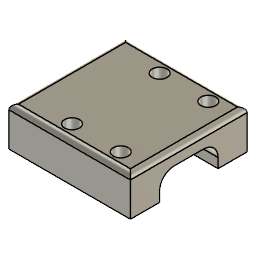
Mouse_Motor_Clamp_Upper_v3 (Autodesk Fusion 360 design; units mm, degrees)
Autodesk Fusion 360 part; units mm, degrees
note: some values were not read from the file. Set by a fixed rule: which sketch regions a step uses.
sketch "Skizze1" plane through (0, 0, 0) normal (0, 0, 1) x (1, 0, 0)
  line L0 (45, -30) -> (45, -50)
  line L1 (45, -50) -> (-45, -50)
  line L2 (-45, -50) -> (-45, -30)
  arc A0 (45, 0) -> (-45, 0) centre (0, 0) ccw
  line L3 (-45, 0) -> (-36, 0)
  line L4 (-36, 0) -> (-36, -30)
  line L5 (-36, -30) -> (-45, -30)
  line L6 (36, 0) -> (36, -30)
  line L7 (36, -30) -> (45, -30)
  line L8 (36, 0) -> (45, 0)
  dimension "d1" = 90
  dimension "d2" = 50
  dimension "d3" = 9
  dimension "d4" = 30
  dimension "d5" = 9
  dimension "d6" = 30
  constraint coincident A0.centre origin
  constraint vertical L0
  constraint horizontal L1
  constraint vertical L2
  constraint horizontal L3
  constraint vertical L4
  constraint horizontal L5
  constraint vertical L6
  constraint horizontal L7
  measures "d1" diameter of A0
  measures "d2" distance of A0.end L1.end
  measures "d3" distance of A0.end L3.end
  measures "d4" distance of A0.end L2.end
  measures "d5" distance of A0.start L6.start
  measures "d6" distance of A0.start L0.start
extrude "Extrusion1" add sketch "Skizze1" along normal blind 1.6 makes body 1
sketch "Skizze2" plane through (0, 0, 1.6) normal (0, 0, 1) x (-1, 0, 0)
  line L0 (-36, 30) -> (-36, 0)
  line L1 (-36, 0) -> (-45, 0)
  arc A0 (-45, 0) -> (45, 0) centre (0, 0) ccw
  line L2 (45, 0) -> (36, 0)
  line L3 (36, 0) -> (36, 30)
  line L4 (36, 30) -> (45, 30)
  line L5 (45, 30) -> (45, 50)
  line L6 (45, 50) -> (-45, 50)
  line L7 (-45, 50) -> (-45, 30)
  line L8 (-45, 30) -> (-36, 30)
  line L9 (36, 15) -> (36, 24)
  line L10 (36, 15) -> (36, 6)
  circle A1 centre (26, 24) radius 1.525
  circle A2 centre (16, 24) radius 1.525
  circle A3 centre (26, 6) radius 1.525
  circle A4 centre (16, 6) radius 1.525
  line L11 (36, 15) -> (36, 9)
  line L12 (36, 9) -> (11, 9)
  line L13 (11, 9) -> (11, 21)
  line L14 (11, 21) -> (36, 21)
  line L15 (36, 21) -> (36, 9)
  line L16 (36, 24) -> (36, 27)
  line L17 (36, 27) -> (4, 27)
  line L18 (4, 27) -> (4, 2)
  line L19 (4, 2) -> (36, 2)
  line L20 (36, 2) -> (36, 27)
  line L21 (-36, 27) -> (-4, 27)
  line L22 (-4, 27) -> (-4, 2)
  line L23 (-4, 2) -> (-36, 2)
  line L24 (-36, 2) -> (-36, 27)
  line L25 (-11, 21) -> (-36, 21)
  line L26 (-36, 21) -> (-11, 21)
  line L27 (-11, 21) -> (-11, 9)
  line L28 (-11, 9) -> (-36, 9)
  line L29 (-36, 9) -> (-36, 21)
  circle A5 centre (-16, 6) radius 1.5
  circle A6 centre (-26, 6) radius 1.5
  circle A7 centre (-16, 24) radius 1.5
  circle A8 centre (-26, 24) radius 1.5
  dimension "d10" = 9
  dimension "d11" = 9
  dimension "d12" = 10
  dimension "d13" = 10
  dimension "d14" = 10
  dimension "d15" = 10
  dimension "d16" = 3.05
  dimension "d17" = 3.05
  dimension "d18" = 3.05
  dimension "d19" = 3.05
  dimension "d20" = 6
  dimension "d21" = 25
  dimension "d22" = 12
  dimension "d23" = 3
  dimension "d24" = 32
  dimension "d25" = 25
  dimension "d30" = 32
  dimension "d31" = 25
  dimension "d32" = 25
  dimension "d33" = 12
  dimension "d35" = 10
  dimension "d37" = 10
  dimension "d38" = 3
  dimension "d39" = 3
  dimension "d40" = 3
  dimension "d41" = 3
  dimension "d42" = 10
  dimension "d43" = 10
  constraint midpoint L3 L9.start
  constraint horizontal L12
  constraint vertical L13
  constraint horizontal L14
  constraint vertical L15
  constraint coincident L3 L16.end
  constraint parallel L3 L16
  constraint horizontal L17
  constraint vertical L18
  constraint horizontal L19
  constraint vertical L20
  constraint coincident L0 L21.start
  constraint horizontal L21
  constraint vertical L22
  constraint horizontal L23
  constraint vertical L24
  constraint perpendicular L22 L25
  constraint horizontal L26
  constraint vertical L27
  constraint horizontal L28
  constraint vertical L29
  measures "d10" distance of L9.start L9.end
  measures "d11" distance of L9.start L10.end
  measures "d12" distance of L10.end A3.centre
  measures "d13" distance of A3.centre A4.centre
  measures "d14" distance of L9.end A1.centre
  measures "d15" distance of A1.centre A2.centre
  measures "d16" diameter of A1
  measures "d17" diameter of A2
  measures "d18" diameter of A3
  measures "d19" diameter of A4
  measures "d20" distance of L9.start L11.end
  measures "d21" distance of L11.end L12.end
  measures "d22" distance of L11.end L14.end
  measures "d23" distance of L9.end L16.end
  measures "d24" distance of L16.end L17.end
  measures "d25" distance of L16.end L19.end
  measures "d30" distance of L21.start L21.end
  measures "d31" distance of L21.start L23.end
  measures "d32" distance of L25.end L25.start
  measures "d33" distance of L25.end L28.end
  measures "d35" distance of A5.centre A6.centre
  measures "d37" distance of A7.centre A8.centre
  measures "d38" diameter of A5
  measures "d39" diameter of A6
  measures "d40" diameter of A7
  measures "d41" diameter of A8
  measures "d42" distance of L24 A6.centre
  measures "d43" distance of L24 A8.centre
extrude "Extrusion2" cut sketch "Skizze2" against normal blind 1.6 contours A1 | A2 | A3 | A4 bodies 1
mirror "Spiegeln1" about plane through (0, 0, 0) normal (1, 0, 0) of "Extrusion2"
extrude "Extrusion3" cut sketch "Skizze2" against normal blind 2 contours L0 L1 A0 L2 L3 L4 L5 L6 L7 L8 L17 L18 L19 L21 L22 L23 bodies 1 makes body 2 at (7.58, -11.953, 0)
extrude "Extrusion12" cut sketch "Skizze2" against normal blind 2 contours L0 L21 L22 L23 L24 L25 L26 L27 L28 | L0 L24 L25 L26 L27 L28 L29 | L3 L9 L10 L12 L13 L14 L16 L17 L18 L19 L20 | L3 L9 L10 L11 L12 L13 L14 L15 L20 bodies 1 2
extrude "Extrusion13" add sketch "Skizze2" along normal blind 7.4 contours L3 L9 L10 L12 L13 L14 L16 L17 L18 L19 L20 | L3 L9 L10 L11 L12 L13 L14 L15 L20 bodies 1 2
extrude "Extrusion14" add 1 faces at (-7.58, -11.953, 9) along direction (0, 0, 1) blind 5 on bodies 1 bodies 1
extrude "Extrusion15" cut sketch "Skizze2" along normal blind 5 contours L3 L9 L10 L11 L12 L13 L14 L15 L20 bodies 1
sketch "Skizze7" plane through (0, 0, 1.6) normal (0, 0, 1) x (-1, 0, 0)
  line L0 (11, 27) -> (4, 27)
  line L1 (4, 27) -> (4, 2)
  line L2 (4, 2) -> (11, 2)
  line L3 (11, 2) -> (11, 27)
  constraint horizontal L0
  constraint vertical L1
  constraint horizontal L2
  constraint vertical L3
extrude "Extrusion16" cut sketch "Skizze7" along normal blind 13 bodies 1
fillet "Abrundung4" radius 3 2 edges at (-23.5, -21, 6.6) (-23.5, -9, 6.6) on bodies 1
sketch "Skizze8" plane through (0, 0, 1.6) normal (0, 0, 1) x (-1, 0, 0)
  line L0 (26, 21) -> (26, 9)
  line L1 (26, 21) -> (36, 21)
  line L2 (36, 21) -> (36, 9)
  line L3 (36, 9) -> (26, 9)
  constraint vertical L0
  constraint horizontal L1
  constraint vertical L2
  constraint horizontal L3
extrude "Extrusion17" cut sketch "Skizze8" along normal blind 5 bodies 1
extrude "Extrusion18" cut 1 faces at (-33.0867, -11.953, 14) along direction (0, 0, -1) blind 4.4 on bodies 1 bodies 1
sketch "Skizze9" plane through (0, 0, 9.6) normal (0, 0, 1) x (-1, 0, 0)
  line L0 (11, 27) -> (11, 2)
  line L1 (11, 2) -> (36, 2)
  line L2 (36, 2) -> (36, 27)
  line L3 (36, 27) -> (11, 27)
  circle A0 centre (26, 24) radius 1.525
  circle A1 centre (16, 24) radius 1.525
  circle A2 centre (16, 6) radius 1.525
  circle A3 centre (26, 6) radius 1.525
  line L4 (11, 2) -> (36, 2)
  line L5 (36, 2) -> (36, 3)
  line L6 (36, 3) -> (11, 3)
  line L7 (11, 3) -> (11, 2)
  dimension "d91" = 25
  constraint horizontal L4
  constraint vertical L5
  constraint horizontal L6
  constraint vertical L7
  constraint coincident L0.end L1.start
  measures "d91" distance of L0.end L1.end
extrude "Extrusion19" cut sketch "Skizze9" against normal blind 20 contours L0 L1 L2 L4 L5 L6 L7 bodies 1
fillet "Abrundung6" radius 1 4 edges at (-36, -15, 9.6) (-23.5, -3, 9.6) (-11, -15, 9.6) (-23.5, -27, 9.6) on bodies 1
